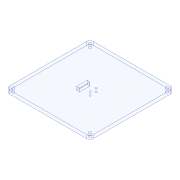
# Autodesk Inventor part: Calibration Arena
Saved by Autodesk Inventor 2020 (Build 240168000, 168)
## iProperties
Created: 2020-08-28
Part Number: Calibration Arena
Material: Generic
Document SubType Name: Modeling
Designer: ferrerx
Density: 1 g/cm^3
Appearance: Clear - Blue
Author: ferrerx
Autodesk Inventor part; units mm, degrees
ref_plane "YZ Plane" through (0, 0, 0) normal (1, 0, 0) x (0, 1, 0)
ref_plane "XZ Plane" through (0, 0, 0) normal (0, 1, 0) x (-1, 0, 0)
ref_plane "XY Plane" through (0, 0, 0) normal (0, 0, 1) x (1, 0, 0)
sketch "Sketch1" plane through (0, 0, 0) normal (0, 1, 0) x (-1, 0, 0)
  line L0 (-60, 60) -> (60, 60)
  line L1 (60, 60) -> (60, -60)
  line L2 (60, -60) -> (-60, -60)
  line L3 (-60, -60) -> (-60, 60)
  line L4 (-60, 60) -> (60, -60) construction
  line L5 (60, 60) -> (-60, -60) construction
  point P0 (0, 0)
  dimension "d0" = 120
  dimension "d1" = 120
  constraints: 12 end point, 2 midpoint, 2 parallel, 1 horizontal, 1 perpendicular
  measures "d0" distance of L1.end L2.end
  measures "d1" distance of L0.end L1.end
extrude "Extrusion1" add sketch "Sketch1" along normal blind 5
sketch "Sketch2" plane through (0, 5, 0) normal (0, 1, 0) x (1, 0, 0)
  line L0 (55, -55) -> (-55, -55) construction
  line L1 (-55, -55) -> (-55, 55) construction
  line L2 (-55, 55) -> (55, 55) construction
  line L3 (55, 55) -> (55, -55) construction
  line L4 (55, -55) -> (-55, 55) construction
  line L5 (-55, -55) -> (55, 55) construction
  circle A0 centre (-55, 55) radius 2
  circle A1 centre (-55, -55) radius 2
  circle A2 centre (55, 55) radius 2
  circle A3 centre (55, -55) radius 2
  point P0 (0, 0)
  dimension "d4" = 110
  dimension "d5" = 110
  dimension "d6" = 4
  dimension "d7" = 4
  dimension "d8" = 4
  dimension "d9" = 4
  constraints: 12 end point, 4 centre point, 4 coincident, 2 midpoint, 2 parallel, 1 horizontal, 1 perpendicular
  measures "d4" distance of L1.end L2.end
  measures "d5" distance of L2.end L0.start
  measures "d6" diameter of A0
  measures "d7" diameter of A3
  measures "d8" diameter of A2
  measures "d9" diameter of A1
extrude "Extrusion2" cut sketch "Sketch2" against normal blind 5
fillet "Fillet1" radius 5 4 edges at (60, 2.5, -60) (60, 2.5, 60) (-60, 2.5, -60) (-60, 2.5, 60)
sketch "Sketch3" plane through (0, 5, 0) normal (0, 1, 0) x (1, 0, 0)
  circle A0 centre (0, 0) radius 7.5
  dimension "d13" = 15
  constraints: 1 centre point, 1 coincident
  measures "d13" diameter of A0
sketch "Sketch4" plane through (0, 5, 0) normal (0, 1, 0) x (1, 0, 0)
  line L0 (-11.5, 7.5) -> (-7.5, 7.5)
  line L1 (-7.5, 7.5) -> (-7.5, -7.5)
  line L2 (-7.5, -7.5) -> (-11.5, -7.5)
  line L3 (-11.5, -7.5) -> (-11.5, 7.5)
  line L4 (-11.5, 7.5) -> (-7.5, -7.5) construction
  line L5 (-7.5, 7.5) -> (-11.5, -7.5) construction
  circle A0 centre (4.5, 4.25) radius 1.25
  circle A1 centre (4.5, -4.25) radius 1.25
  point P0 (0, 0)
  point P1 (-9.5, 0)
  dimension "d14" = 4
  dimension "d15" = 15
  dimension "d16" = 9.5
  dimension "d17" = 14
  dimension "d18" = 14
  dimension "d19" = 2.5
  dimension "d20" = 2.5
  dimension "d21" = 8.5
  dimension "d22" = 4.25
  constraints: 12 end point, 2 centre point, 2 midpoint, 2 parallel, 1 horizontal, 1 perpendicular
  measures "d14" distance of L1.end L2.end
  measures "d15" distance of L2.end L0.start
  measures "d16" distance of point (0, 0) point (-9.5, 0)
  measures "d17" horizontal distance of point (-9.5, 0) A0.centre
  measures "d18" horizontal distance of point (-9.5, 0) A1.centre
  measures "d19" diameter of A1
  measures "d20" diameter of A0
  measures "d21" distance of A0.centre A1.centre
  measures "d22" vertical distance of point (-9.5, 0) A1.centre
extrude "Extrusion3" cut sketch "Sketch4" against normal blind 10
body "Solid1"
